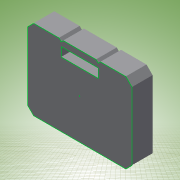
# Autodesk Inventor part: Divider_box
Saved by Autodesk Inventor 2017 (Build 210142000, 142)
## iProperties
Created: 2018-06-04
Part Number: Divider_box
Material: Generic
Document SubType Name: Modeling
Designer: Spark Electronics
Density: 1 g/cm^3
Appearance: Default
Author: Spark Electronics
Autodesk Inventor part; units mm, degrees
ref_plane "YZ Plane" through (0, 0, 0) normal (1, 0, 0) x (0, 1, 0)
ref_plane "XZ Plane" through (0, 0, 0) normal (0, 1, 0) x (-1, 0, 0)
ref_plane "XY Plane" through (0, 0, 0) normal (0, 0, 1) x (1, 0, 0)
sketch "Sketch1" plane through (0, 0, 0) normal (0, 0, 1) x (1, 0, 0)
  line L0 (215.9, -165.1) -> (-215.9, -165.1)
  line L1 (-215.9, -165.1) -> (-215.9, 165.1)
  line L2 (215.9, 165.1) -> (215.9, -165.1)
  line L3 (215.9, -165.1) -> (-215.9, 165.1) construction
  line L4 (-215.9, -165.1) -> (215.9, 165.1) construction
  line L5 (76.2, 101.6) -> (-76.4881, 101.6)
  line L6 (-76.2, 191.0151) -> (76.2, 101.6) construction
  line L7 (76.2, 191.0151) -> (-76.4881, 101.6) construction
  line L8 (66.0896, 101.6) -> (-66.0896, 101.6)
  line L9 (-67.8456, 164.5323) -> (67.5575, 164.5323)
  line L10 (76.2, 139.1323) -> (-76.4881, 139.1323)
  line L11 (-76.4881, 155.8898) -> (-67.8456, 164.5323)
  line L12 (-0.144, 139.1323) -> (-0.144, 146.3921)
  line L13 (76.2, 155.8898) -> (67.5575, 164.5323)
  line L14 (-215.9, 165.1) -> (-85.6983, 165.1)
  line L15 (-67.8456, 164.5323) -> (67.5575, 164.5323)
  line L16 (85.4102, 165.1) -> (215.9, 165.1)
  line L17 (76.2, 139.1323) -> (76.2, 101.6)
  line L18 (-76.4881, 101.6) -> (-76.4881, 139.1323)
  line L19 (-76.4881, 155.8898) -> (-85.6983, 165.1)
  line L20 (76.2, 155.8898) -> (85.4102, 165.1)
  point P0 (0, 0)
  point P1 (-0.072, 146.3498)
  dimension "d0" = 431.8
  dimension "d1" = 330.2
  dimension "d7" = 266.7
  dimension "d11" = 25.4
  dimension "d12" = 45
  constraints: 42 end point, 6 parallel, 3 horizontal, 3 midpoint, 3 point on line, 2 perpendicular, 2 symmetric about line
  measures "d0" distance of L1.end L2.start
  measures "d1" distance of L0.end L1.end
  measures "d7" distance between parallel lines of L0 L5
  measures "d11" distance between parallel lines of L9 L10
  measures "d12" angle of L14 L19
extrude "Extrusion1" add sketch "Sketch1" along normal blind 85.725
chamfer "Chamfer1" distance 25.4 angle 45 4 edges at (215.9, 165.1, 42.8625) (215.9, -165.1, 42.8625) (-215.9, -165.1, 42.8625) (-215.9, 165.1, 42.8625)
sketch "Sketch2" plane through (0, 0, 85.725) normal (0, 0, 1) x (1, 0, 0)
  line L0 (76.2, 139.1323) -> (76.2, 101.6) projected
  line L1 (76.2, 101.6) -> (-76.4881, 101.6) projected
  line L2 (-76.4881, 101.6) -> (-76.4881, 139.1323) projected
  line L3 (-215.9, 139.7) -> (-190.5, 165.1) projected
  line L4 (-215.9, 139.7) -> (-215.9, -139.7) projected
  line L5 (-190.5, -165.1) -> (-215.9, -139.7) projected
  line L6 (-190.5, -165.1) -> (190.5, -165.1) projected
  line L7 (215.9, -139.7) -> (190.5, -165.1) projected
  line L8 (215.9, -139.7) -> (215.9, 139.7) projected
  line L9 (190.5, 165.1) -> (215.9, 139.7) projected
  line L10 (190.5, 165.1) -> (85.4102, 165.1) projected
  line L11 (85.4102, 165.1) -> (76.2, 155.8898) projected
  line L12 (76.2, 155.8898) -> (67.5575, 164.5323) projected
  line L13 (67.5575, 164.5323) -> (-67.8456, 164.5323) projected
  line L14 (-67.8456, 164.5323) -> (-76.4881, 155.8898) projected
  line L15 (-76.4881, 155.8898) -> (-85.6983, 165.1) projected
  line L16 (-85.6983, 165.1) -> (-190.5, 165.1) projected
  line L17 (-76.4881, 139.1323) -> (76.2, 139.1323) projected
  line L18 (-76.4881, 139.1323) -> (-76.4881, 155.8898)
  line L19 (76.2, 139.1323) -> (76.2, 155.8898)
  point P0 (0, 0)
  constraints: 4 end point, 1 parallel, 1 perpendicular
extrude "Extrusion2" cut sketch "Sketch2" against normal blind 30.1625 contours L17 L18 L14 L13 L12 L19
sketch "Sketch3" plane through (0, 0, 0) normal (0, 0, -1) x (-1, 0, 0)
  line L0 (76.4881, 139.1323) -> (76.4881, 101.6) projected
  line L1 (76.4881, 101.6) -> (-76.2, 101.6) projected
  line L2 (-76.2, 101.6) -> (-76.2, 139.1323) projected
  line L3 (-76.2, 139.1323) -> (76.4881, 139.1323) projected
  line L4 (190.5, 165.1) -> (215.9, 139.7) projected
  line L5 (85.6983, 165.1) -> (190.5, 165.1) projected
  line L6 (76.4881, 155.8898) -> (85.6983, 165.1) projected
  line L7 (67.8456, 164.5323) -> (76.4881, 155.8898) projected
  line L8 (-67.5575, 164.5323) -> (67.8456, 164.5323) projected
  line L9 (-76.2, 155.8898) -> (-67.5575, 164.5323) projected
  line L10 (-85.4102, 165.1) -> (-76.2, 155.8898) projected
  line L11 (-190.5, 165.1) -> (-85.4102, 165.1) projected
  line L12 (-215.9, 139.7) -> (-190.5, 165.1) projected
  line L13 (-215.9, -139.7) -> (-215.9, 139.7) projected
  line L14 (-190.5, -165.1) -> (-215.9, -139.7) projected
  line L15 (190.5, -165.1) -> (-190.5, -165.1) projected
  line L16 (215.9, -139.7) -> (190.5, -165.1) projected
  line L17 (215.9, 139.7) -> (215.9, -139.7) projected
  line L18 (-76.2, 139.1323) -> (76.4881, 139.1323) projected
  line L19 (-76.2, 139.1323) -> (-76.2, 155.8898)
  line L20 (76.4881, 101.6) -> (76.4881, 155.8898) projected
  line L21 (76.4881, 139.1323) -> (76.4881, 155.8898)
  point P0 (0, 0)
  constraints: 4 end point, 1 perpendicular, 1 vertical
extrude "Extrusion3" cut sketch "Sketch3" against normal blind 30.1625 contours L3 L19 L9 L8 L7 L20
chamfer "Chamfer2" distance 3.175 angle 45 4 edges at (-0.144, 139.1323, 55.5625) (-0.144, 139.1323, 30.1625) (-0.144, 164.5323, 55.5625) (-0.144, 164.5323, 30.1625)
body "Solid1"
